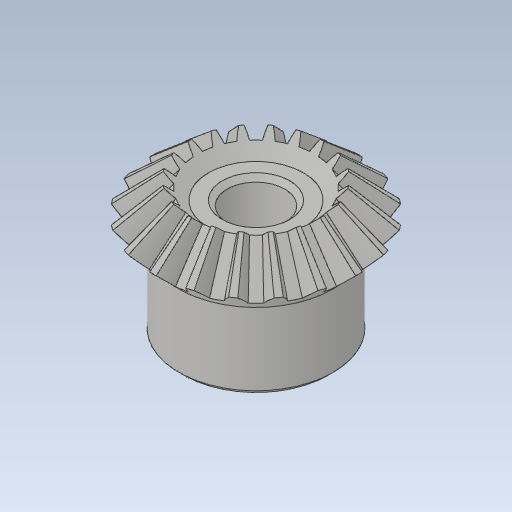
# Autodesk Inventor part: PM1-201_On
Saved by Autodesk Inventor 2024 (Build 280153000, 153)
## iProperties
Created: 2023-09-12
Part Number: PM1-201_On
Material: Generic
Catalog Web Link: www.cadenas.de
Description: PM-
Vendor: KHK
Document SubType Name: Modeling
Designer: psAdmin
Manufacturer: KHK
Mass: 2.33933 g
Surface Area: 15.3806 cm^2
Volume: 2.33933 cm^3
Density: 1 g/cm^3
Appearance: PSOLRGB-175-175-175
Category: PARTsolutions
Company: KHK
PSOL_IDENT_0: {$CADENAS_DATA/23d-libs/khk/miter_gears/pm.prj},169 {VTYP=3D},{NB=PM1-201_On},{LINA=PM1-20},{NN=PM},
PSOL_IDENT_1: {DATE=06.10.2022 23:14:45},{GEOMDATE=25.04.2019 06:31:30},{VERSION=},{LINEID=20},{WBVAR=COMBINATION,
PSOL_IDENT_2: TOOTH},{WBNUMERIC=}  {NB=PM1-201_On},{LINA=PM1-20},{KT=DUMMY},{CN=PM1-20},{COMBINATION=1},{M=1.00},{
PSOL_IDENT_3: Z=20},{A=6},{B=16},{C=20},{D=21.41},{E=20},{F=13.95},{G=10.71},{H=8.0},{I=12},{J=5},{K=9.86},{L=49.8
PSOL_IDENT_4: 0},{S=B3},{PN=PM1-20},{WMF=B3003.WMF},{X=0.5},{Y=0.5},{TOOTH=On}
NB: PM1-201_On
NN: PM
NBSYN: $CN.$COMBINATION._$TOOTH.
LINA: PM1-20
CATALOG: KHK
CN: PM1-20
COMBINATION: Single
M: 1
Z: 20
A: 6
B: 16
C: 20
D: 21.41
E: 20
F: 13.95
G: 10.71
H: 8
I: 12
J: 5
K: 9.86
L: 49.8
S: B3
PN: PM1-20
WMF: B3003.WMF
X: 0.5
Y: 0.5
TOOTH: On
SUPPLIER: KHK
ARTICLENO: PM1-201_On
BOMINFO: PM1-20
CREATOR: CADENAS GmbH
Title: PM1-20
Author: Cadenas PARTsolutions
Autodesk Inventor part; units mm, degrees
sketch "Sketch_4" plane through (0, -12, 0) normal (0, 1, 0) x (1, 0, 0)
  arc A0 (-0.3583, 14.2515) -> (-1.0036, 9.0909) centre (13.0701, 9.9515) ccw
  arc A1 (-1.0036, 9.0909) -> (-1.8547, 8.9561) centre (0, 0) ccw
  arc A2 (-1.8547, 8.9561) -> (-4.0632, 13.6647) centre (-15.5055, 5.4255) ccw
  arc A3 (-4.0632, 13.6647) -> (-4.7447, 13.4432) centre (0, 0) ccw
  arc A4 (-4.7447, 13.4432) -> (-3.7638, 8.3358) centre (9.3552, 13.5033) ccw
  arc A5 (-3.7638, 8.3358) -> (-4.5315, 7.9446) centre (0, 0) ccw
  arc A6 (-4.5315, 7.9446) -> (-8.087, 11.7403) centre (-16.4232, 0.3685) ccw
  arc A7 (-8.087, 11.7403) -> (-8.6666, 11.3191) centre (0, 0) ccw
  arc A8 (-8.6666, 11.3191) -> (-6.1555, 6.7648) centre (4.7246, 15.7333) ccw
  arc A9 (-6.1555, 6.7648) -> (-6.7648, 6.1555) centre (0, 0) ccw
  arc A10 (-6.7648, 6.1555) -> (-11.3191, 8.6666) centre (-15.7333, -4.7246) ccw
  arc A11 (-11.3191, 8.6666) -> (-11.7403, 8.087) centre (0, 0) ccw
  arc A12 (-11.7403, 8.087) -> (-7.9446, 4.5315) centre (-0.3685, 16.4232) ccw
  arc A13 (-7.9446, 4.5315) -> (-8.3358, 3.7638) centre (0, 0) ccw
  arc A14 (-8.3358, 3.7638) -> (-13.4432, 4.7447) centre (-13.5033, -9.3552) ccw
  arc A15 (-13.4432, 4.7447) -> (-13.6647, 4.0632) centre (0, 0) ccw
  arc A16 (-13.6647, 4.0632) -> (-8.9561, 1.8547) centre (-5.4255, 15.5055) ccw
  arc A17 (-8.9561, 1.8547) -> (-9.0909, 1.0036) centre (0, 0) ccw
  arc A18 (-9.0909, 1.0036) -> (-14.2515, 0.3583) centre (-9.9515, -13.0701) ccw
  arc A19 (-14.2515, 0.3583) -> (-14.2515, -0.3583) centre (0, 0) ccw
  arc A20 (-14.2515, -0.3583) -> (-9.0909, -1.0036) centre (-9.9515, 13.0701) ccw
  arc A21 (-9.0909, -1.0036) -> (-8.9561, -1.8547) centre (0, 0) ccw
  arc A22 (-8.9561, -1.8547) -> (-13.6647, -4.0632) centre (-5.4255, -15.5055) ccw
  arc A23 (-13.6647, -4.0632) -> (-13.4432, -4.7447) centre (0, 0) ccw
  arc A24 (-13.4432, -4.7447) -> (-8.3358, -3.7638) centre (-13.5033, 9.3552) ccw
  arc A25 (-8.3358, -3.7638) -> (-7.9446, -4.5315) centre (0, 0) ccw
  arc A26 (-7.9446, -4.5315) -> (-11.7403, -8.087) centre (-0.3685, -16.4232) ccw
  arc A27 (-11.7403, -8.087) -> (-11.3191, -8.6666) centre (0, 0) ccw
  arc A28 (-11.3191, -8.6666) -> (-6.7648, -6.1555) centre (-15.7333, 4.7246) ccw
  arc A29 (-6.7648, -6.1555) -> (-6.1555, -6.7648) centre (0, 0) ccw
  arc A30 (-6.1555, -6.7648) -> (-8.6666, -11.3191) centre (4.7246, -15.7333) ccw
  arc A31 (-8.6666, -11.3191) -> (-8.087, -11.7403) centre (0, 0) ccw
  arc A32 (-8.087, -11.7403) -> (-4.5315, -7.9446) centre (-16.4232, -0.3685) ccw
  arc A33 (-4.5315, -7.9446) -> (-3.7638, -8.3358) centre (0, 0) ccw
  arc A34 (-3.7638, -8.3358) -> (-4.7447, -13.4432) centre (9.3552, -13.5033) ccw
  arc A35 (-4.7447, -13.4432) -> (-4.0632, -13.6647) centre (0, 0) ccw
  arc A36 (-4.0632, -13.6647) -> (-1.8547, -8.9561) centre (-15.5055, -5.4255) ccw
  arc A37 (-1.8547, -8.9561) -> (-1.0036, -9.0909) centre (0, 0) ccw
  arc A38 (-1.0036, -9.0909) -> (-0.3583, -14.2515) centre (13.0701, -9.9515) ccw
  arc A39 (-0.3583, -14.2515) -> (0.3583, -14.2515) centre (0, 0) ccw
  arc A40 (0.3583, -14.2515) -> (1.0036, -9.0909) centre (-13.0701, -9.9515) ccw
  arc A41 (1.0036, -9.0909) -> (1.8547, -8.9561) centre (0, 0) ccw
  arc A42 (1.8547, -8.9561) -> (4.0632, -13.6647) centre (15.5055, -5.4255) ccw
  arc A43 (4.0632, -13.6647) -> (4.7447, -13.4432) centre (0, 0) ccw
  arc A44 (4.7447, -13.4432) -> (3.7638, -8.3358) centre (-9.3552, -13.5033) ccw
  arc A45 (3.7638, -8.3358) -> (4.5315, -7.9446) centre (0, 0) ccw
  arc A46 (4.5315, -7.9446) -> (8.087, -11.7403) centre (16.4232, -0.3685) ccw
  arc A47 (8.087, -11.7403) -> (8.6666, -11.3191) centre (0, 0) ccw
  arc A48 (8.6666, -11.3191) -> (6.1555, -6.7648) centre (-4.7246, -15.7333) ccw
  arc A49 (6.1555, -6.7648) -> (6.7648, -6.1555) centre (0, 0) ccw
  arc A50 (6.7648, -6.1555) -> (11.3191, -8.6666) centre (15.7333, 4.7246) ccw
  arc A51 (11.3191, -8.6666) -> (11.7403, -8.087) centre (0, 0) ccw
  arc A52 (11.7403, -8.087) -> (7.9446, -4.5315) centre (0.3685, -16.4232) ccw
  arc A53 (7.9446, -4.5315) -> (8.3358, -3.7638) centre (0, 0) ccw
  arc A54 (8.3358, -3.7638) -> (13.4432, -4.7447) centre (13.5033, 9.3552) ccw
  arc A55 (13.4432, -4.7447) -> (13.6647, -4.0632) centre (0, 0) ccw
  arc A56 (13.6647, -4.0632) -> (8.9561, -1.8547) centre (5.4255, -15.5055) ccw
  arc A57 (8.9561, -1.8547) -> (9.0909, -1.0036) centre (0, 0) ccw
  arc A58 (9.0909, -1.0036) -> (14.2515, -0.3583) centre (9.9515, 13.0701) ccw
  arc A59 (14.2515, -0.3583) -> (14.2515, 0.3583) centre (0, 0) ccw
  arc A60 (14.2515, 0.3583) -> (9.0909, 1.0036) centre (9.9515, -13.0701) ccw
  arc A61 (9.0909, 1.0036) -> (8.9561, 1.8547) centre (0, 0) ccw
  arc A62 (8.9561, 1.8547) -> (13.6647, 4.0632) centre (5.4255, 15.5055) ccw
  arc A63 (13.6647, 4.0632) -> (13.4432, 4.7447) centre (0, 0) ccw
  arc A64 (13.4432, 4.7447) -> (8.3358, 3.7638) centre (13.5033, -9.3552) ccw
  arc A65 (8.3358, 3.7638) -> (7.9446, 4.5315) centre (0, 0) ccw
  arc A66 (7.9446, 4.5315) -> (11.7403, 8.087) centre (0.3685, 16.4232) ccw
  arc A67 (11.7403, 8.087) -> (11.3191, 8.6666) centre (0, 0) ccw
  arc A68 (11.3191, 8.6666) -> (6.7648, 6.1555) centre (15.7333, -4.7246) ccw
  arc A69 (6.7648, 6.1555) -> (6.1555, 6.7648) centre (0, 0) ccw
  arc A70 (6.1555, 6.7648) -> (8.6666, 11.3191) centre (-4.7246, 15.7333) ccw
  arc A71 (8.6666, 11.3191) -> (8.087, 11.7403) centre (0, 0) ccw
  arc A72 (8.087, 11.7403) -> (4.5315, 7.9446) centre (16.4232, 0.3685) ccw
  arc A73 (4.5315, 7.9446) -> (3.7638, 8.3358) centre (0, 0) ccw
  arc A74 (3.7638, 8.3358) -> (4.7447, 13.4432) centre (-9.3552, 13.5033) ccw
  arc A75 (4.7447, 13.4432) -> (4.0632, 13.6647) centre (0, 0) ccw
  arc A76 (4.0632, 13.6647) -> (1.8547, 8.9561) centre (15.5055, 5.4255) ccw
  arc A77 (1.8547, 8.9561) -> (1.0036, 9.0909) centre (0, 0) ccw
  arc A78 (1.0036, 9.0909) -> (0.3583, 14.2515) centre (-13.0701, 9.9515) ccw
  arc A79 (0.3583, 14.2515) -> (-0.3583, 14.2515) centre (0, 0) ccw
  constraints: 160 point on circle, 80 centre point
sketch "Sketch_5" plane through (0, -6.05, 0) normal (0, 1, 0) x (1, 0, 0)
  arc A0 (-0.1354, 7.1843) -> (-0.399, 3.6144) centre (13.6807, 4.3695) ccw
  arc A1 (-0.399, 3.6144) -> (-0.7374, 3.5608) centre (0, 0) ccw
  arc A2 (-0.7374, 3.5608) -> (-2.0913, 6.8746) centre (-14.3614, -0.072) ccw
  arc A3 (-2.0913, 6.8746) -> (-2.3489, 6.7908) centre (0, 0) ccw
  arc A4 (-2.3489, 6.7908) -> (-1.4964, 3.3142) centre (11.6609, 8.3832) ccw
  arc A5 (-1.4964, 3.3142) -> (-1.8017, 3.1587) centre (0, 0) ccw
  arc A6 (-1.8017, 3.1587) -> (-4.1133, 5.8918) centre (-13.6363, -4.5064) ccw
  arc A7 (-4.1133, 5.8918) -> (-4.3324, 5.7326) centre (0, 0) ccw
  arc A8 (-4.3324, 5.7326) -> (-2.4473, 2.6896) centre (8.4996, 11.5763) ccw
  arc A9 (-2.4473, 2.6896) -> (-2.6896, 2.4473) centre (0, 0) ccw
  arc A10 (-2.6896, 2.4473) -> (-5.7326, 4.3324) centre (-11.5763, -8.4996) ccw
  arc A11 (-5.7326, 4.3324) -> (-5.8918, 4.1133) centre (0, 0) ccw
  arc A12 (-5.8918, 4.1133) -> (-3.1587, 1.8017) centre (4.5064, 13.6363) ccw
  arc A13 (-3.1587, 1.8017) -> (-3.3142, 1.4964) centre (0, 0) ccw
  arc A14 (-3.3142, 1.4964) -> (-6.7908, 2.3489) centre (-8.3832, -11.6609) ccw
  arc A15 (-6.7908, 2.3489) -> (-6.8746, 2.0913) centre (0, 0) ccw
  arc A16 (-6.8746, 2.0913) -> (-3.5608, 0.7374) centre (0.072, 14.3614) ccw
  arc A17 (-3.5608, 0.7374) -> (-3.6144, 0.399) centre (0, 0) ccw
  arc A18 (-3.6144, 0.399) -> (-7.1843, 0.1354) centre (-4.3695, -13.6807) ccw
  arc A19 (-7.1843, 0.1354) -> (-7.1843, -0.1354) centre (0, 0) ccw
  arc A20 (-7.1843, -0.1354) -> (-3.6144, -0.399) centre (-4.3695, 13.6807) ccw
  arc A21 (-3.6144, -0.399) -> (-3.5608, -0.7374) centre (0, 0) ccw
  arc A22 (-3.5608, -0.7374) -> (-6.8746, -2.0913) centre (0.072, -14.3614) ccw
  arc A23 (-6.8746, -2.0913) -> (-6.7908, -2.3489) centre (0, 0) ccw
  arc A24 (-6.7908, -2.3489) -> (-3.3142, -1.4964) centre (-8.3832, 11.6609) ccw
  arc A25 (-3.3142, -1.4964) -> (-3.1587, -1.8017) centre (0, 0) ccw
  arc A26 (-3.1587, -1.8017) -> (-5.8918, -4.1133) centre (4.5064, -13.6363) ccw
  arc A27 (-5.8918, -4.1133) -> (-5.7326, -4.3324) centre (0, 0) ccw
  arc A28 (-5.7326, -4.3324) -> (-2.6896, -2.4473) centre (-11.5763, 8.4996) ccw
  arc A29 (-2.6896, -2.4473) -> (-2.4473, -2.6896) centre (0, 0) ccw
  arc A30 (-2.4473, -2.6896) -> (-4.3324, -5.7326) centre (8.4996, -11.5763) ccw
  arc A31 (-4.3324, -5.7326) -> (-4.1133, -5.8918) centre (0, 0) ccw
  arc A32 (-4.1133, -5.8918) -> (-1.8017, -3.1587) centre (-13.6363, 4.5064) ccw
  arc A33 (-1.8017, -3.1587) -> (-1.4964, -3.3142) centre (0, 0) ccw
  arc A34 (-1.4964, -3.3142) -> (-2.3489, -6.7908) centre (11.6609, -8.3832) ccw
  arc A35 (-2.3489, -6.7908) -> (-2.0913, -6.8746) centre (0, 0) ccw
  arc A36 (-2.0913, -6.8746) -> (-0.7374, -3.5608) centre (-14.3614, 0.072) ccw
  arc A37 (-0.7374, -3.5608) -> (-0.399, -3.6144) centre (0, 0) ccw
  arc A38 (-0.399, -3.6144) -> (-0.1354, -7.1843) centre (13.6807, -4.3695) ccw
  arc A39 (-0.1354, -7.1843) -> (0.1354, -7.1843) centre (0, 0) ccw
  arc A40 (0.1354, -7.1843) -> (0.399, -3.6144) centre (-13.6807, -4.3695) ccw
  arc A41 (0.399, -3.6144) -> (0.7374, -3.5608) centre (0, 0) ccw
  arc A42 (0.7374, -3.5608) -> (2.0913, -6.8746) centre (14.3614, 0.072) ccw
  arc A43 (2.0913, -6.8746) -> (2.3489, -6.7908) centre (0, 0) ccw
  arc A44 (2.3489, -6.7908) -> (1.4964, -3.3142) centre (-11.6609, -8.3832) ccw
  arc A45 (1.4964, -3.3142) -> (1.8017, -3.1587) centre (0, 0) ccw
  arc A46 (1.8017, -3.1587) -> (4.1133, -5.8918) centre (13.6363, 4.5064) ccw
  arc A47 (4.1133, -5.8918) -> (4.3324, -5.7326) centre (0, 0) ccw
  arc A48 (4.3324, -5.7326) -> (2.4473, -2.6896) centre (-8.4996, -11.5763) ccw
  arc A49 (2.4473, -2.6896) -> (2.6896, -2.4473) centre (0, 0) ccw
  arc A50 (2.6896, -2.4473) -> (5.7326, -4.3324) centre (11.5763, 8.4996) ccw
  arc A51 (5.7326, -4.3324) -> (5.8918, -4.1133) centre (0, 0) ccw
  arc A52 (5.8918, -4.1133) -> (3.1587, -1.8017) centre (-4.5064, -13.6363) ccw
  arc A53 (3.1587, -1.8017) -> (3.3142, -1.4964) centre (0, 0) ccw
  arc A54 (3.3142, -1.4964) -> (6.7908, -2.3489) centre (8.3832, 11.6609) ccw
  arc A55 (6.7908, -2.3489) -> (6.8746, -2.0913) centre (0, 0) ccw
  arc A56 (6.8746, -2.0913) -> (3.5608, -0.7374) centre (-0.072, -14.3614) ccw
  arc A57 (3.5608, -0.7374) -> (3.6144, -0.399) centre (0, 0) ccw
  arc A58 (3.6144, -0.399) -> (7.1843, -0.1354) centre (4.3695, 13.6807) ccw
  arc A59 (7.1843, -0.1354) -> (7.1843, 0.1354) centre (0, 0) ccw
  arc A60 (7.1843, 0.1354) -> (3.6144, 0.399) centre (4.3695, -13.6807) ccw
  arc A61 (3.6144, 0.399) -> (3.5608, 0.7374) centre (0, 0) ccw
  arc A62 (3.5608, 0.7374) -> (6.8746, 2.0913) centre (-0.072, 14.3614) ccw
  arc A63 (6.8746, 2.0913) -> (6.7908, 2.3489) centre (0, 0) ccw
  arc A64 (6.7908, 2.3489) -> (3.3142, 1.4964) centre (8.3832, -11.6609) ccw
  arc A65 (3.3142, 1.4964) -> (3.1587, 1.8017) centre (0, 0) ccw
  arc A66 (3.1587, 1.8017) -> (5.8918, 4.1133) centre (-4.5064, 13.6363) ccw
  arc A67 (5.8918, 4.1133) -> (5.7326, 4.3324) centre (0, 0) ccw
  arc A68 (5.7326, 4.3324) -> (2.6896, 2.4473) centre (11.5763, -8.4996) ccw
  arc A69 (2.6896, 2.4473) -> (2.4473, 2.6896) centre (0, 0) ccw
  arc A70 (2.4473, 2.6896) -> (4.3324, 5.7326) centre (-8.4996, 11.5763) ccw
  arc A71 (4.3324, 5.7326) -> (4.1133, 5.8918) centre (0, 0) ccw
  arc A72 (4.1133, 5.8918) -> (1.8017, 3.1587) centre (13.6363, -4.5064) ccw
  arc A73 (1.8017, 3.1587) -> (1.4964, 3.3142) centre (0, 0) ccw
  arc A74 (1.4964, 3.3142) -> (2.3489, 6.7908) centre (-11.6609, 8.3832) ccw
  arc A75 (2.3489, 6.7908) -> (2.0913, 6.8746) centre (0, 0) ccw
  arc A76 (2.0913, 6.8746) -> (0.7374, 3.5608) centre (14.3614, -0.072) ccw
  arc A77 (0.7374, 3.5608) -> (0.399, 3.6144) centre (0, 0) ccw
  arc A78 (0.399, 3.6144) -> (0.1354, 7.1843) centre (-13.6807, 4.3695) ccw
  arc A79 (0.1354, 7.1843) -> (-0.1354, 7.1843) centre (0, 0) ccw
  constraints: 160 point on circle, 80 centre point
loft "Loft1" add profiles "Sketch_4", "Sketch_5"
sketch "Sketch_6" plane through (0, 0, 0) normal (0, 0, 1) x (1, 0, 0)
  line L0 (0, -20) -> (0, -8)
  line L1 (0, -8) -> (4.93, -8)
  line L2 (4.93, -8) -> (6.0517, -6.873)
  line L3 (6.0517, -6.873) -> (9.2912, -10.7064)
  line L4 (9.2912, -10.7064) -> (8, -12)
  line L5 (8, -12) -> (8, -19.5)
  line L6 (8, -19.5) -> (7.5, -20)
  line L7 (7.5, -20) -> (0, -20)
  line L8 (0, -20) -> (0, -8)
  constraints: 18 end point
revolve "Revolution1" add sketch "Sketch_6" angle 360 about axis through (0, -20, 0) along (0, -1, 0)
sketch "Sketch_7" plane through (0, 0, 0) normal (0, 0, 1) x (1, 0, 0)
  line L0 (0, -20) -> (0, 0)
  line L1 (0, 0) -> (21.41, 0)
  line L2 (21.41, 0) -> (21.41, -12)
  line L3 (21.41, -12) -> (8, -12)
  line L4 (8, -12) -> (10.705, -9.29)
  line L5 (10.705, -9.29) -> (6.871, -6.05)
  line L6 (6.871, -6.05) -> (4.93, -8)
  line L7 (4.93, -8) -> (3.5, -8)
  line L8 (3.5, -8) -> (3, -8.5)
  line L9 (3, -8.5) -> (3, -19.5)
  line L10 (3, -19.5) -> (3.5, -20)
  line L11 (3.5, -20) -> (0, -20)
  line L12 (0, -20) -> (0, 0)
  constraints: 26 end point
revolve "Revolution2" cut sketch "Sketch_7" angle 360 about axis through (0, -20, 0) along (0, -1, 0)
ref_plane "IP2_XY" through (0, 0, 0) normal (0, 0, 1) x (1, 0, 0)
ref_plane "IP2_YZ" through (0, 0, 0) normal (1, 0, 0) x (0, 1, 0)
ref_plane "IP2_ZX" through (0, 0, 0) normal (0, 1, 0) x (0, 0, 1)
ref_plane "pm_XY" through (0, 0, 0) normal (0, 1, 0) x (1, 0, 0)
ref_plane "pm_YZ" through (0, 0, 0) normal (1, 0, 0) x (0, 0, -1)
ref_plane "pm_ZX" through (0, 0, 0) normal (0, 0, -1) x (0, 1, 0)
body "Solid1"
